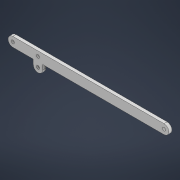
# Autodesk Inventor part: Wing
Saved by Autodesk Inventor 2021 (Build 250183000, 183)
## iProperties
Created: 2021-01-28
Part Number: Wing
Material: Generic
Document SubType Name: Modeling
Designer: argon
Density: 1 g/cm^3
Appearance: Default
Author: argon
Autodesk Inventor part; units mm, degrees
ref_plane "YZ Plane" through (0, 0, 0) normal (1, 0, 0) x (0, 1, 0)
ref_plane "XZ Plane" through (0, 0, 0) normal (0, 1, 0) x (-1, 0, 0)
ref_plane "XY Plane" through (0, 0, 0) normal (0, 0, 1) x (1, 0, 0)
sketch "Sketch1" plane through (0, 0, 0) normal (0, 0, 1) x (1, 0, 0)
  circle A0 centre (-48, 0) radius 1
  circle A1 centre (48, 0) radius 1
  line L0 (-48, 0) -> (0, 0) construction
  line L1 (0, 0) -> (48, 0) construction
  line L2 (-48, 3) -> (48, 3)
  line L3 (-48, -3) -> (48, -3)
  line L4 (0, 3) -> (0, -3) construction
  arc A2 (-48, 3) -> (-48, -3) centre (-48, 0) ccw
  arc A3 (48, -3) -> (48, 3) centre (48, 0) ccw
  circle A4 centre (-32, 0) radius 1
  circle A5 centre (-32, -6) radius 3
  line L5 (-35, -6) -> (-35, -3)
  line L6 (-29, -6) -> (-29, -3)
  circle A6 centre (-32, -6) radius 1
  point P0 (-48, -1)
  dimension "d0" = 2
  dimension "d1" = 2
  dimension "d2" = 48
  dimension "d5" = 16
  constraints: 14 end point, 6 centre point, 6 point on circle, 4 coincident, 4 vertical alignment, 3 horizontal, 3 midpoint, 3 point on line, 2 equal length, 2 equal radius, 2 perpendicular, 2 tangent, 1 collinear, 1 vertical, 4 other
  measures "d1" distance of L3.start point (-48, -1)
  measures "d2" distance of L0.start L0.end
  measures "d5" distance of A4.centre L0.start
extrude "Extrusion1" add sketch "Sketch1" along normal blind 2
body "Solid1"
